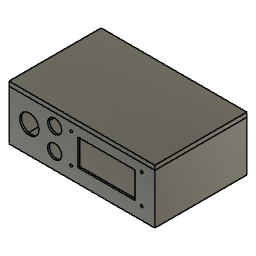
SparkFun DataLogger casing v4 (Autodesk Fusion 360 design; units mm, degrees)
Autodesk Fusion 360 part; units mm, degrees
note: some values were not read from the file. Set by a fixed rule: which sketch regions a step uses.
sketch "Sketch1" plane through (0, 0, 0) normal (0, 0, 1) x (1, 0, 0)
  line L0 (81.15, 50.5) -> (-81.15, 50.5)
  line L1 (-81.15, 50.5) -> (-81.15, -50.5)
  line L2 (-81.15, -50.5) -> (81.15, -50.5)
  line L3 (81.15, -50.5) -> (81.15, 50.5)
  line L4 (81.15, 50.5) -> (-81.15, -50.5) construction
  line L5 (-81.15, 50.5) -> (81.15, -50.5) construction
  line L6 (83.15, 52.5) -> (-83.15, 52.5)
  line L7 (-83.15, 52.5) -> (-83.15, -52.5)
  line L8 (-83.15, -52.5) -> (83.15, -52.5)
  line L9 (83.15, -52.5) -> (83.15, 52.5)
  line L10 (83.15, 52.5) -> (-83.15, -52.5) construction
  line L11 (-83.15, 52.5) -> (83.15, -52.5) construction
  dimension "d1" = 162.3
  dimension "d2" = 101
  dimension "d3" = 166.3
  dimension "d4" = 105
  constraint horizontal L0
  constraint perpendicular L0 L1
  constraint parallel L0 L2
  constraint parallel L1 L3
  constraint coincident L4 origin
  constraint coincident L5 origin
  constraint horizontal L6
  constraint perpendicular L6 L7
  constraint parallel L6 L8
  constraint parallel L7 L9
  constraint coincident L10 origin
  constraint coincident L11 origin
  measures "d1" distance of L1.end L2.end
  measures "d2" distance of L0.end L1.end
  measures "d3" distance of L7.end L8.end
  measures "d4" distance of L6.end L7.end
extrude "Extrude1" add sketch "Sketch1" along normal blind 2 contours L0 L1 L2 L3 | L6 L7 L8 L9 makes body 1
extrude "Extrude2" add sketch "Sketch1" along normal blind 52 bodies 1
sketch "Sketch2" plane through (0, -52.5, 0) normal (0, -1, 0) x (1, 0, 0)
  line L0 (-83.15, 0) -> (83.15, 0)
  line L1 (83.15, 0) -> (83.15, 52)
  line L2 (83.15, 52) -> (-83.15, 52)
  line L3 (-83.15, 52) -> (-83.15, 0)
  circle A0 centre (-44, 26) radius 11
  line L4 (-15.6464, 46.2394) -> (71.6464, 46.2394)
  line L5 (71.6464, 46.2394) -> (71.6464, 5.7606)
  line L6 (71.6464, 5.7606) -> (-15.6464, 5.7606)
  line L7 (-15.6464, 5.7606) -> (-15.6464, 46.2394)
  line L8 (-15.6464, 46.2394) -> (71.6464, 5.7606) construction
  line L9 (71.6464, 46.2394) -> (-15.6464, 5.7606) construction
  line L10 (-4.4815, 41.0368) -> (60.4815, 41.0368)
  line L11 (60.4815, 41.0368) -> (60.4815, 10.9632)
  line L12 (60.4815, 10.9632) -> (-4.4815, 10.9632)
  line L13 (-4.4815, 10.9632) -> (-4.4815, 41.0368)
  line L14 (-4.4815, 41.0368) -> (60.4815, 10.9632) construction
  line L15 (60.4815, 41.0368) -> (-4.4815, 10.9632) construction
  line L16 (0, 26) -> (-83.15, 26)
  line L17 (0, 26) -> (83.15, 26)
  line L18 (-15.6464, 46.2394) -> (-12.2464, 46.2394)
  line L19 (-12.2464, 46.2394) -> (-12.2464, 42.8394)
  circle A1 centre (-12.2464, 42.8394) radius 1.5
  circle A2 centre (68.2464, 42.8394) radius 1.5
  circle A3 centre (-12.2464, 9.1606) radius 1.5
  circle A4 centre (68.2464, 9.1606) radius 1.5
  point P0 (28, 26)
  point P1 (28, 26)
  dimension "d10" = 22
  dimension "d21" = 3.4
  dimension "d22" = 3.4
  dimension "d23" = 3
  constraint horizontal L4
  constraint perpendicular L4 L5
  constraint parallel L4 L6
  constraint parallel L5 L7
  constraint coincident L8 P1
  constraint coincident L9 P1
  constraint horizontal L10
  constraint perpendicular L10 L11
  constraint parallel L10 L12
  constraint parallel L11 L13
  constraint coincident L14 P1
  constraint coincident L15 P1
  constraint coincident P1 P0
  constraint midpoint L3 L16.end
  constraint midpoint L1 L17.end
  constraint perpendicular L7 L18
  constraint perpendicular L18 L19
  constraint coincident L19.end A1.centre
  constraint symmetric L17 A1 A3
  constraint symmetric L17 A2 A4
  measures "d10" diameter of A0
  measures "d21" distance of L4.start L18.end
  measures "d22" distance of L18.end L19.end
  measures "d23" diameter of A1
extrude "Extrude3" cut sketch "Sketch2" against normal blind 5 contours A0 L16 | A0 L16 | L10 L11 L13 L16 L17 | L11 L12 L13 L16 L17 bodies 1
extrude "Extrude4" add 1 faces at (-27.7167, -17.5, 0) along direction (0, 0, -1) blind 5 on bodies 1 bodies 1
extrude "Extrude5" cut 1 faces at (-27.05, 16.8333, 2) along direction (0, 0, -1) blind 5 on bodies 1 bodies 1
move_body "Move1" bodies 1 to x (1, 0, 0) y (0, 1, 0) z (0, 0, 1) at (0, 0, 5)
extrude "Extrude6" cut sketch "Sketch2" against normal blind 28 contours A1 | A2 | A3 | A4 bodies 1
move_face "MoveFace1" to x (1, 0, 0) y (0, 1, 0) z (0, 0, 1) at (0, 0, 5) 4 faces at (-10.7538, -51.8333, 9.0113) (-10.8642, -51.8333, 43.422) (69.2938, -51.8333, 43.9132) (67.7687, -51.8333, 7.7387) on bodies 1
sketch "Sketch3" plane through (0, 0, 2) normal (0, 0, 1) x (-1, 0, 0)
  line L0 (-81.15, -50.5) -> (81.15, -50.5)
  line L1 (81.15, -50.5) -> (81.15, 50.5)
  line L2 (81.15, 50.5) -> (-81.15, 50.5)
  line L3 (-81.15, 50.5) -> (-81.15, -50.5)
  line L4 (-72.2, -43.15) -> (72.2, 43.15) construction
  line L5 (72.2, -43.15) -> (-72.2, 43.15) construction
  circle A0 centre (73.7, -44.65) radius 1.5
  circle A1 centre (-73.7, -44.65) radius 1.5
  circle A2 centre (-73.7, 44.65) radius 1.5
  circle A3 centre (76.3, 44.65) radius 1.5
  circle A4 centre (76.3, 44.65) radius 3.5
  circle A5 centre (73.7, -44.65) radius 3.5
  circle A6 centre (-73.7, -44.65) radius 3.5
  circle A7 centre (-73.7, 44.65) radius 3.5
  dimension "d26" = 144.4
  dimension "d27" = 86.3
  dimension "d28" = 1.5
  dimension "d29" = 1.5
  dimension "d30" = 1.5
  dimension "d32" = 1.5
  dimension "d33" = 7
  dimension "d34" = 7
  dimension "d35" = 7
  dimension "d36" = 7
  constraint coincident L4 origin
  constraint coincident L5 origin
  constraint concentric A3 A4
  constraint concentric A0 A5
  constraint concentric A1 A6
  constraint concentric A2 A7
  measures "d26" distance of L4.end L5.end
  measures "d27" distance of L5.start L4.end
  measures "d28" radius of A0
  measures "d29" radius of A1
  measures "d30" radius of A2
  measures "d32" radius of A3
  measures "d33" diameter of A4
  measures "d34" diameter of A5
  measures "d35" diameter of A6
  measures "d36" diameter of A7
extrude "Extrude7" add sketch "Sketch3" along normal blind 5 contours A4 | A5 | A6 | A7 bodies 1
sketch "Sketch4" plane through (0, 0, 57) normal (0, 0, 1) x (-1, 0, 0)
  line L0 (-81.15, -50.5) -> (-81.15, 50.5)
  line L1 (-81.15, 50.5) -> (81.15, 50.5)
  line L2 (81.15, 50.5) -> (81.15, -50.5)
  line L3 (81.15, -50.5) -> (-81.15, -50.5)
  line L4 (-83.15, 52.5) -> (-83.15, -52.5)
  line L5 (-83.15, -52.5) -> (83.15, -52.5)
  line L6 (83.15, -52.5) -> (83.15, 52.5)
  line L7 (83.15, 52.5) -> (-83.15, 52.5)
extrude "Extrude8" add sketch "Sketch4" against normal blind 3 separate body contours L0 L1 L2 L3 makes body 2
extrude "Extrude9" add 1 faces at (27.05, -16.8333, 57) along direction (0, 0, 1) blind 5 separate body on bodies 2 makes body 3
move_face "OffsetFaces1" offset 2 4 faces at (27.05, -50.5, 58.6667) (81.15, 16.8333, 60.3333) (-27.05, 50.5, 58.6667) (-81.15, -16.8333, 60.3333) on bodies 3
combine "Combine1" operation add target body 3 tool bodies 2
move_face "OffsetFaces2" offset -0.125 4 faces at (-81.15, -16.8333, 56) (27.05, -50.5, 56) (81.15, 16.8333, 56) (-27.05, 50.5, 56) on bodies 3
sketch "Sketch5" plane through (0, -52.5, 0) normal (0, -1, 0) x (1, 0, 0)
  circle A0 centre (-12.2464, 14.1606) radius 1.5
  circle A1 centre (68.2464, 14.1606) radius 1.5
  circle A2 centre (-12.2464, 47.8394) radius 1.5
  circle A3 centre (68.2464, 47.8394) radius 1.5
  circle A4 centre (-44, 31) radius 11
  line L0 (60.4815, 46.0368) -> (60.4815, 15.9632)
  line L1 (60.4815, 15.9632) -> (-4.4815, 15.9632)
  line L2 (-4.4815, 15.9632) -> (-4.4815, 46.0368)
  line L3 (-4.4815, 46.0368) -> (60.4815, 46.0368)
  line L4 (83.15, 0) -> (83.15, 57)
  line L5 (83.15, 57) -> (-83.15, 57)
  line L6 (-83.15, 57) -> (-83.15, 0)
  line L7 (-83.15, 0) -> (83.15, 0)
  circle A5 centre (-70.1333, 43.5) radius 8
  circle A6 centre (-70.1333, 18.5) radius 8
  dimension "d47" = 16
  measures "d47" diameter of A5
extrude "Extrude10" cut sketch "Sketch5" against normal blind 3 contours A5 | A6 bodies 1
move_face "MoveFace2" to x (1, 0, 0) y (0, 1, 0) z (0, 0, 1) at (44, 0, 0) 2 faces at (-62.1432, -51.1667, 18.1012) (-62.1432, -51.1667, 43.1012) on bodies 1
move_face "MoveFace3" to x (1, 0, 0) y (0, 1, 0) z (0, 0, 1) at (-16, 0, 0) 1 faces at (-33.0547, -51.8333, 32.0952) on bodies 1
move_face "MoveFace4" to x (1, 0, 0) y (0, 1, 0) z (0, 0, 1) at (-5, 0, 0) 2 faces at (-18.173, -51.8333, 17.7035) (-18.173, -51.8333, 42.7035) on bodies 1
equation "d1 = 157 mm + 3.3 mm + 2 mm"
equation "d3 = 162.30000 mm + 4 mm"
equation "d4 = 101.00000 mm + 4 mm"
equation "d7 = 2 mm + 50 mm"
equation "d44 = ( -0.25 / 2 ) * 1 mm"
